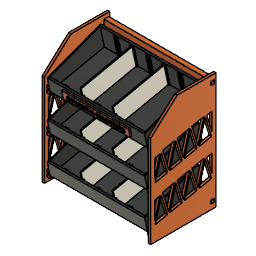
binstack-print-assembly.f3z (Autodesk Fusion 360 design; units mm, degrees)
part number: 2026-08-18-20-33-43-765
part number: 2026-08-18-20-33-45-073
part number: 2026-08-18-20-33-45-486
part number: 2026-08-18-20-33-45-986
part number: 2026-08-18-20-33-46-975
part number: 2026-08-18-20-33-47-360
part number: 2026-08-18-20-33-47-431
Autodesk Fusion 360 part; units mm, degrees
sketch "Sketch1" plane through (0, 0, 0) normal (1, 0, 0) x (0, 0, -1) in component "Боковина левая"
  line L0 (0, 15) -> (0, 150)
  line L1 (0, 150) -> (-240, 150)
  line L2 (-240, 150) -> (-240, 70)
  line L3 (-240, 70) -> (-190, 15)
  line L4 (-190, 15) -> (0, 15)
extrude "Extrude1" add sketch "Sketch1" along normal blind 5 from surface at 3 makes body 1 in component "Боковина левая"
sketch "Sketch2" plane through (0, 0, 0) normal (1, 0, 0) x (0, 0, -1) in component "Боковина левая"
  line L0 (-9, 20) -> (-35.5696, 145)
  line L1 (-35.5696, 145) -> (-41.5696, 145)
  line L2 (-41.5696, 145) -> (-15, 20)
  line L3 (-15, 20) -> (-9, 20)
extrude "Extrude2" add sketch "Sketch2" along normal blind 6 from surface at 8 separate body makes body 2 in component "Боковина левая"
sketch "Sketch3" plane through (0, 0, 0) normal (1, 0, 0) x (0, 0, -1) in component "Боковина левая"
  line L0 (-18.2, 20) -> (-44.7696, 145)
  line L1 (-44.7696, 145) -> (-49.7696, 145)
  line L2 (-49.7696, 145) -> (-23.2, 20)
  line L3 (-23.2, 20) -> (-18.2, 20)
extrude "Extrude3" add sketch "Sketch3" along normal blind 6 from surface at 8 separate body makes body 3 in component "Боковина левая"
sketch "Sketch4" plane through (0, 0, 0) normal (1, 0, 0) x (0, 0, -1) in component "Боковина левая"
  line L0 (-16.2753, 26) -> (-17.2753, 28)
  line L1 (-17.2753, 28) -> (-18.3381, 31)
  line L2 (-18.3381, 31) -> (-17.7632, 33)
  line L3 (-17.7632, 33) -> (-16.2753, 26)
extrude "Extrude4" add sketch "Sketch4" along normal blind 6 from surface at 8 separate body makes body 4 in component "Боковина левая"
sketch "Sketch5" plane through (0, 0, 0) normal (1, 0, 0) x (0, 0, -1) in component "Боковина левая"
  line L0 (-84, 20) -> (-110.5696, 145)
  line L1 (-110.5696, 145) -> (-116.5696, 145)
  line L2 (-116.5696, 145) -> (-90, 20)
  line L3 (-90, 20) -> (-84, 20)
extrude "Extrude5" add sketch "Sketch5" along normal blind 6 from surface at 8 separate body makes body 5 in component "Боковина левая"
sketch "Sketch6" plane through (0, 0, 0) normal (1, 0, 0) x (0, 0, -1) in component "Боковина левая"
  line L0 (-93.2, 20) -> (-119.7696, 145)
  line L1 (-119.7696, 145) -> (-124.7696, 145)
  line L2 (-124.7696, 145) -> (-98.2, 20)
  line L3 (-98.2, 20) -> (-93.2, 20)
extrude "Extrude6" add sketch "Sketch6" along normal blind 6 from surface at 8 separate body makes body 6 in component "Боковина левая"
sketch "Sketch7" plane through (0, 0, 0) normal (1, 0, 0) x (0, 0, -1) in component "Боковина левая"
  line L0 (-91.2753, 26) -> (-92.2753, 28)
  line L1 (-92.2753, 28) -> (-93.3381, 31)
  line L2 (-93.3381, 31) -> (-92.7632, 33)
  line L3 (-92.7632, 33) -> (-91.2753, 26)
extrude "Extrude7" add sketch "Sketch7" along normal blind 6 from surface at 8 separate body makes body 7 in component "Боковина левая"
sketch "Sketch8" plane through (0, 0, 0) normal (1, 0, 0) x (0, 0, -1) in component "Боковина левая"
  line L0 (-159, 20) -> (-185.5696, 145)
  line L1 (-185.5696, 145) -> (-191.5696, 145)
  line L2 (-191.5696, 145) -> (-165, 20)
  line L3 (-165, 20) -> (-159, 20)
extrude "Extrude8" add sketch "Sketch8" along normal blind 6 from surface at 8 separate body makes body 8 in component "Боковина левая"
sketch "Sketch9" plane through (0, 0, 0) normal (1, 0, 0) x (0, 0, -1) in component "Боковина левая"
  line L0 (-168.2, 20) -> (-194.7696, 145)
  line L1 (-194.7696, 145) -> (-199.7696, 145)
  line L2 (-199.7696, 145) -> (-173.2, 20)
  line L3 (-173.2, 20) -> (-168.2, 20)
extrude "Extrude9" add sketch "Sketch9" along normal blind 6 from surface at 8 separate body makes body 9 in component "Боковина левая"
sketch "Sketch10" plane through (0, 0, 0) normal (1, 0, 0) x (0, 0, -1) in component "Боковина левая"
  line L0 (-166.2753, 26) -> (-167.2753, 28)
  line L1 (-167.2753, 28) -> (-168.3381, 31)
  line L2 (-168.3381, 31) -> (-167.7632, 33)
  line L3 (-167.7632, 33) -> (-166.2753, 26)
extrude "Extrude10" add sketch "Sketch10" along normal blind 6 from surface at 8 separate body makes body 10 in component "Боковина левая"
combine "Combine1" operation add target body 1 tool bodies 2 3 4 5 6 7 8 9 10 in component "Боковина левая"
sketch "Sketch11" plane through (0, 0, 0) normal (1, 0, 0) x (0, 0, -1) in component "Боковина левая"
  line L0 (-10.5, 139.5) -> (-10.5, 146.5)
  line L1 (-10.5, 146.5) -> (-17.5, 146.5)
  line L2 (-17.5, 146.5) -> (-17.5, 139.5)
  line L3 (-17.5, 139.5) -> (-10.5, 139.5)
extrude "Extrude11" cut sketch "Sketch11" along normal blind 30 from surface at -2 bodies 1 in component "Боковина левая"
sketch "Sketch12" plane through (0, 0, 0) normal (1, 0, 0) x (0, 0, -1) in component "Боковина левая"
  line L0 (-222.5, 139.5) -> (-222.5, 146.5)
  line L1 (-222.5, 146.5) -> (-229.5, 146.5)
  line L2 (-229.5, 146.5) -> (-229.5, 139.5)
  line L3 (-229.5, 139.5) -> (-222.5, 139.5)
extrude "Extrude12" cut sketch "Sketch12" along normal blind 30 from surface at -2 bodies 1 in component "Боковина левая"
sketch "Sketch13" plane through (0, 0, 0) normal (1, 0, 0) x (0, 0, -1) in component "Боковина левая"
  line L0 (-31.2766, 24.6534) -> (-36.5785, 49.5966)
  line L1 (-36.5785, 49.5966) -> (-77.4649, 37.125)
  line L2 (-77.4649, 37.125) -> (-31.2766, 24.6534)
  line L3 (-37.7065, 54.9034) -> (-43.0083, 79.8466)
  line L4 (-43.0083, 79.8466) -> (-83.8948, 67.375)
  line L5 (-83.8948, 67.375) -> (-37.7065, 54.9034)
  line L6 (-44.1363, 85.1534) -> (-49.4382, 110.0966)
  line L7 (-49.4382, 110.0966) -> (-90.3246, 97.625)
  line L8 (-90.3246, 97.625) -> (-44.1363, 85.1534)
  line L9 (-50.5662, 115.4034) -> (-55.868, 140.3466)
  line L10 (-55.868, 140.3466) -> (-96.7545, 127.875)
  line L11 (-96.7545, 127.875) -> (-50.5662, 115.4034)
  line L12 (-81.1165, 39.7784) -> (-86.4183, 64.7216)
  line L13 (-86.4183, 64.7216) -> (-40.23, 52.25)
  line L14 (-40.23, 52.25) -> (-81.1165, 39.7784)
  line L15 (-87.5463, 70.0284) -> (-92.8482, 94.9716)
  line L16 (-92.8482, 94.9716) -> (-46.6599, 82.5)
  line L17 (-46.6599, 82.5) -> (-87.5463, 70.0284)
  line L18 (-93.9761, 100.2784) -> (-99.278, 125.2216)
  line L19 (-99.278, 125.2216) -> (-53.0897, 112.75)
  line L20 (-53.0897, 112.75) -> (-93.9761, 100.2784)
  line L21 (-38.7844, 23.5511) -> (-75.34, 23.5511)
  line L22 (-75.34, 23.5511) -> (-77.5658, 34.0228)
  line L23 (-77.5658, 34.0228) -> (-38.7844, 23.5511)
  line L24 (-63.8444, 141.4489) -> (-100.3999, 141.4489)
  line L25 (-100.3999, 141.4489) -> (-98.1741, 130.9772)
  line L26 (-98.1741, 130.9772) -> (-63.8444, 141.4489)
  line L27 (-106.2766, 24.6534) -> (-111.5785, 49.5966)
  line L28 (-111.5785, 49.5966) -> (-152.4649, 37.125)
  line L29 (-152.4649, 37.125) -> (-106.2766, 24.6534)
  line L30 (-112.7065, 54.9034) -> (-118.0083, 79.8466)
  line L31 (-118.0083, 79.8466) -> (-158.8948, 67.375)
  line L32 (-158.8948, 67.375) -> (-112.7065, 54.9034)
  line L33 (-119.1363, 85.1534) -> (-124.4382, 110.0966)
  line L34 (-124.4382, 110.0966) -> (-165.3246, 97.625)
  line L35 (-165.3246, 97.625) -> (-119.1363, 85.1534)
  line L36 (-125.5662, 115.4034) -> (-130.868, 140.3466)
  line L37 (-130.868, 140.3466) -> (-171.7545, 127.875)
  line L38 (-171.7545, 127.875) -> (-125.5662, 115.4034)
  line L39 (-156.1165, 39.7784) -> (-161.4183, 64.7216)
  line L40 (-161.4183, 64.7216) -> (-115.23, 52.25)
  line L41 (-115.23, 52.25) -> (-156.1165, 39.7784)
  line L42 (-162.5463, 70.0284) -> (-167.8482, 94.9716)
  line L43 (-167.8482, 94.9716) -> (-121.6599, 82.5)
  line L44 (-121.6599, 82.5) -> (-162.5463, 70.0284)
  line L45 (-168.9761, 100.2784) -> (-174.278, 125.2216)
  line L46 (-174.278, 125.2216) -> (-128.0897, 112.75)
  line L47 (-128.0897, 112.75) -> (-168.9761, 100.2784)
  line L48 (-113.7844, 23.5511) -> (-150.34, 23.5511)
  line L49 (-150.34, 23.5511) -> (-152.5658, 34.0228)
  line L50 (-152.5658, 34.0228) -> (-113.7844, 23.5511)
  line L51 (-138.8444, 141.4489) -> (-175.3999, 141.4489)
  line L52 (-175.3999, 141.4489) -> (-173.1741, 130.9772)
  line L53 (-173.1741, 130.9772) -> (-138.8444, 141.4489)
extrude "Extrude13" cut sketch "Sketch13" along normal blind 9 from surface at 1 bodies 1 in component "Боковина левая"
sketch "Sketch1 (2)" plane through (0, 0, 0) normal (1, 0, 0) x (0, 0, -1) in component "Боковина правая"
  line L0 (0, 15) -> (0, 150)
  line L1 (0, 150) -> (-240, 150)
  line L2 (-240, 150) -> (-240, 70)
  line L3 (-240, 70) -> (-190, 15)
  line L4 (-190, 15) -> (0, 15)
extrude "Extrude1'" add sketch "Sketch1 (2)" along normal blind 5 from surface at 6 separate body makes body 11 in component "Боковина правая"
sketch "Sketch2 (2)" plane through (0, 0, 0) normal (1, 0, 0) x (0, 0, -1) in component "Боковина правая"
  line L0 (-9, 20) -> (-35.5696, 145)
  line L1 (-35.5696, 145) -> (-41.5696, 145)
  line L2 (-41.5696, 145) -> (-15, 20)
  line L3 (-15, 20) -> (-9, 20)
extrude "Extrude2'" add sketch "Sketch2 (2)" along normal blind 6 separate body makes body 12 in component "Боковина правая"
sketch "Sketch3 (2)" plane through (0, 0, 0) normal (1, 0, 0) x (0, 0, -1) in component "Боковина правая"
  line L0 (-18.2, 20) -> (-44.7696, 145)
  line L1 (-44.7696, 145) -> (-49.7696, 145)
  line L2 (-49.7696, 145) -> (-23.2, 20)
  line L3 (-23.2, 20) -> (-18.2, 20)
extrude "Extrude3'" add sketch "Sketch3 (2)" along normal blind 6 separate body makes body 13 in component "Боковина правая"
sketch "Sketch4 (2)" plane through (0, 0, 0) normal (1, 0, 0) x (0, 0, -1) in component "Боковина правая"
  line L0 (-16.2753, 26) -> (-17.2753, 28)
  line L1 (-17.2753, 28) -> (-18.3381, 31)
  line L2 (-18.3381, 31) -> (-17.7632, 33)
  line L3 (-17.7632, 33) -> (-16.2753, 26)
extrude "Extrude4'" add sketch "Sketch4 (2)" along normal blind 6 separate body makes body 14 in component "Боковина правая"
sketch "Sketch5 (2)" plane through (0, 0, 0) normal (1, 0, 0) x (0, 0, -1) in component "Боковина правая"
  line L0 (-84, 20) -> (-110.5696, 145)
  line L1 (-110.5696, 145) -> (-116.5696, 145)
  line L2 (-116.5696, 145) -> (-90, 20)
  line L3 (-90, 20) -> (-84, 20)
extrude "Extrude5'" add sketch "Sketch5 (2)" along normal blind 6 separate body makes body 15 in component "Боковина правая"
sketch "Sketch6 (2)" plane through (0, 0, 0) normal (1, 0, 0) x (0, 0, -1) in component "Боковина правая"
  line L0 (-93.2, 20) -> (-119.7696, 145)
  line L1 (-119.7696, 145) -> (-124.7696, 145)
  line L2 (-124.7696, 145) -> (-98.2, 20)
  line L3 (-98.2, 20) -> (-93.2, 20)
extrude "Extrude6'" add sketch "Sketch6 (2)" along normal blind 6 separate body makes body 16 in component "Боковина правая"
sketch "Sketch7 (2)" plane through (0, 0, 0) normal (1, 0, 0) x (0, 0, -1) in component "Боковина правая"
  line L0 (-91.2753, 26) -> (-92.2753, 28)
  line L1 (-92.2753, 28) -> (-93.3381, 31)
  line L2 (-93.3381, 31) -> (-92.7632, 33)
  line L3 (-92.7632, 33) -> (-91.2753, 26)
extrude "Extrude7'" add sketch "Sketch7 (2)" along normal blind 6 separate body makes body 17 in component "Боковина правая"
sketch "Sketch8 (2)" plane through (0, 0, 0) normal (1, 0, 0) x (0, 0, -1) in component "Боковина правая"
  line L0 (-159, 20) -> (-185.5696, 145)
  line L1 (-185.5696, 145) -> (-191.5696, 145)
  line L2 (-191.5696, 145) -> (-165, 20)
  line L3 (-165, 20) -> (-159, 20)
extrude "Extrude8'" add sketch "Sketch8 (2)" along normal blind 6 separate body makes body 18 in component "Боковина правая"
sketch "Sketch9 (2)" plane through (0, 0, 0) normal (1, 0, 0) x (0, 0, -1) in component "Боковина правая"
  line L0 (-168.2, 20) -> (-194.7696, 145)
  line L1 (-194.7696, 145) -> (-199.7696, 145)
  line L2 (-199.7696, 145) -> (-173.2, 20)
  line L3 (-173.2, 20) -> (-168.2, 20)
extrude "Extrude9'" add sketch "Sketch9 (2)" along normal blind 6 separate body makes body 19 in component "Боковина правая"
sketch "Sketch10 (2)" plane through (0, 0, 0) normal (1, 0, 0) x (0, 0, -1) in component "Боковина правая"
  line L0 (-166.2753, 26) -> (-167.2753, 28)
  line L1 (-167.2753, 28) -> (-168.3381, 31)
  line L2 (-168.3381, 31) -> (-167.7632, 33)
  line L3 (-167.7632, 33) -> (-166.2753, 26)
extrude "Extrude10'" add sketch "Sketch10 (2)" along normal blind 6 separate body makes body 20 in component "Боковина правая"
combine "Combine1'" operation add target body 11 tool bodies 12 13 14 15 16 17 18 19 20 in component "Боковина правая"
sketch "Sketch11 (2)" plane through (0, 0, 0) normal (1, 0, 0) x (0, 0, -1) in component "Боковина правая"
  line L0 (-10.5, 139.5) -> (-10.5, 146.5)
  line L1 (-10.5, 146.5) -> (-17.5, 146.5)
  line L2 (-17.5, 146.5) -> (-17.5, 139.5)
  line L3 (-17.5, 139.5) -> (-10.5, 139.5)
extrude "Extrude11'" cut sketch "Sketch11 (2)" along normal blind 30 from surface at -2 bodies 11 in component "Боковина правая"
sketch "Sketch12 (2)" plane through (0, 0, 0) normal (1, 0, 0) x (0, 0, -1) in component "Боковина правая"
  line L0 (-222.5, 139.5) -> (-222.5, 146.5)
  line L1 (-222.5, 146.5) -> (-229.5, 146.5)
  line L2 (-229.5, 146.5) -> (-229.5, 139.5)
  line L3 (-229.5, 139.5) -> (-222.5, 139.5)
extrude "Extrude12'" cut sketch "Sketch12 (2)" along normal blind 30 from surface at -2 bodies 11 in component "Боковина правая"
sketch "Sketch13 (2)" plane through (0, 0, 0) normal (1, 0, 0) x (0, 0, -1) in component "Боковина правая"
  line L0 (-31.2766, 24.6534) -> (-36.5785, 49.5966)
  line L1 (-36.5785, 49.5966) -> (-77.4649, 37.125)
  line L2 (-77.4649, 37.125) -> (-31.2766, 24.6534)
  line L3 (-37.7065, 54.9034) -> (-43.0083, 79.8466)
  line L4 (-43.0083, 79.8466) -> (-83.8948, 67.375)
  line L5 (-83.8948, 67.375) -> (-37.7065, 54.9034)
  line L6 (-44.1363, 85.1534) -> (-49.4382, 110.0966)
  line L7 (-49.4382, 110.0966) -> (-90.3246, 97.625)
  line L8 (-90.3246, 97.625) -> (-44.1363, 85.1534)
  line L9 (-50.5662, 115.4034) -> (-55.868, 140.3466)
  line L10 (-55.868, 140.3466) -> (-96.7545, 127.875)
  line L11 (-96.7545, 127.875) -> (-50.5662, 115.4034)
  line L12 (-81.1165, 39.7784) -> (-86.4183, 64.7216)
  line L13 (-86.4183, 64.7216) -> (-40.23, 52.25)
  line L14 (-40.23, 52.25) -> (-81.1165, 39.7784)
  line L15 (-87.5463, 70.0284) -> (-92.8482, 94.9716)
  line L16 (-92.8482, 94.9716) -> (-46.6599, 82.5)
  line L17 (-46.6599, 82.5) -> (-87.5463, 70.0284)
  line L18 (-93.9761, 100.2784) -> (-99.278, 125.2216)
  line L19 (-99.278, 125.2216) -> (-53.0897, 112.75)
  line L20 (-53.0897, 112.75) -> (-93.9761, 100.2784)
  line L21 (-38.7844, 23.5511) -> (-75.34, 23.5511)
  line L22 (-75.34, 23.5511) -> (-77.5658, 34.0228)
  line L23 (-77.5658, 34.0228) -> (-38.7844, 23.5511)
  line L24 (-63.8444, 141.4489) -> (-100.3999, 141.4489)
  line L25 (-100.3999, 141.4489) -> (-98.1741, 130.9772)
  line L26 (-98.1741, 130.9772) -> (-63.8444, 141.4489)
  line L27 (-106.2766, 24.6534) -> (-111.5785, 49.5966)
  line L28 (-111.5785, 49.5966) -> (-152.4649, 37.125)
  line L29 (-152.4649, 37.125) -> (-106.2766, 24.6534)
  line L30 (-112.7065, 54.9034) -> (-118.0083, 79.8466)
  line L31 (-118.0083, 79.8466) -> (-158.8948, 67.375)
  line L32 (-158.8948, 67.375) -> (-112.7065, 54.9034)
  line L33 (-119.1363, 85.1534) -> (-124.4382, 110.0966)
  line L34 (-124.4382, 110.0966) -> (-165.3246, 97.625)
  line L35 (-165.3246, 97.625) -> (-119.1363, 85.1534)
  line L36 (-125.5662, 115.4034) -> (-130.868, 140.3466)
  line L37 (-130.868, 140.3466) -> (-171.7545, 127.875)
  line L38 (-171.7545, 127.875) -> (-125.5662, 115.4034)
  line L39 (-156.1165, 39.7784) -> (-161.4183, 64.7216)
  line L40 (-161.4183, 64.7216) -> (-115.23, 52.25)
  line L41 (-115.23, 52.25) -> (-156.1165, 39.7784)
  line L42 (-162.5463, 70.0284) -> (-167.8482, 94.9716)
  line L43 (-167.8482, 94.9716) -> (-121.6599, 82.5)
  line L44 (-121.6599, 82.5) -> (-162.5463, 70.0284)
  line L45 (-168.9761, 100.2784) -> (-174.278, 125.2216)
  line L46 (-174.278, 125.2216) -> (-128.0897, 112.75)
  line L47 (-128.0897, 112.75) -> (-168.9761, 100.2784)
  line L48 (-113.7844, 23.5511) -> (-150.34, 23.5511)
  line L49 (-150.34, 23.5511) -> (-152.5658, 34.0228)
  line L50 (-152.5658, 34.0228) -> (-113.7844, 23.5511)
  line L51 (-138.8444, 141.4489) -> (-175.3999, 141.4489)
  line L52 (-175.3999, 141.4489) -> (-173.1741, 130.9772)
  line L53 (-173.1741, 130.9772) -> (-138.8444, 141.4489)
extrude "Extrude13'" cut sketch "Sketch13 (2)" along normal blind 9 from surface at 4 bodies 11 in component "Боковина правая"
sketch "Sketch1 (3)" plane through (0, 0, 0) normal (0, 0, 1) x (1, 0, 0) in component "Лоток"
  line L0 (-6, 0) -> (207, 0)
  line L1 (207, 0) -> (207, 117)
  line L2 (207, 117) -> (-6, 117)
  line L3 (-6, 117) -> (-6, 0)
extrude "Extrude1''" add sketch "Sketch1 (3)" along normal blind 2.4 separate body makes body 21 in component "Лоток"
sketch "Sketch2 (3)" plane through (0, 0, 0) normal (0, 0, 1) x (1, 0, 0) in component "Лоток"
  line L0 (0, 0) -> (201, 0)
  line L1 (201, 0) -> (201, 4)
  line L2 (201, 4) -> (0, 4)
  line L3 (0, 4) -> (0, 0)
extrude "Extrude2''" add sketch "Sketch2 (3)" along normal blind 28 separate body makes body 22 in component "Лоток"
sketch "Sketch3 (3)" plane through (0, 0, 0) normal (0, 0, 1) x (1, 0, 0) in component "Лоток"
  line L0 (0, 113) -> (201, 113)
  line L1 (201, 113) -> (201, 117)
  line L2 (201, 117) -> (0, 117)
  line L3 (0, 117) -> (0, 113)
extrude "Extrude3''" add sketch "Sketch3 (3)" along normal blind 45 separate body makes body 23 in component "Лоток"
sketch "Sketch4 (3)" plane through (0, 0, 0) normal (1, 0, 0) x (0, 0, -1) in component "Лоток"
  line L0 (0, 0) -> (0, 117)
  line L1 (0, 117) -> (-45, 117)
  line L2 (-45, 117) -> (-28, 0)
  line L3 (-28, 0) -> (0, 0)
extrude "Extrude4''" add sketch "Sketch4 (3)" along normal blind 2 separate body makes body 24 in component "Лоток"
sketch "Sketch5 (3)" plane through (0, 0, 0) normal (1, 0, 0) x (0, 0, -1) in component "Лоток"
  line L0 (0, 0) -> (0, 117)
  line L1 (0, 117) -> (-45, 117)
  line L2 (-45, 117) -> (-28, 0)
  line L3 (-28, 0) -> (0, 0)
extrude "Extrude5''" add sketch "Sketch5 (3)" along normal blind 2 from surface at 199 separate body makes body 25 in component "Лоток"
sketch "Sketch6 (3)" plane through (0, 0, 0) normal (0, 0, 1) x (1, 0, 0) in component "Лоток"
  line L0 (31.4, 4) -> (33.4, 4)
  line L1 (33.4, 4) -> (33.4, 6)
  line L2 (33.4, 6) -> (31.4, 6)
  line L3 (31.4, 6) -> (31.4, 4)
extrude "Extrude6''" add sketch "Sketch6 (3)" along normal blind 25.6 from surface at 2.4 separate body makes body 26 in component "Лоток"
sketch "Sketch7 (3)" plane through (0, 0, 0) normal (0, 0, 1) x (1, 0, 0) in component "Лоток"
  line L0 (31.4, 111) -> (33.4, 111)
  line L1 (33.4, 111) -> (33.4, 113)
  line L2 (33.4, 113) -> (31.4, 113)
  line L3 (31.4, 113) -> (31.4, 111)
extrude "Extrude7''" add sketch "Sketch7 (3)" along normal blind 42.6 from surface at 2.4 separate body makes body 27 in component "Лоток"
sketch "Sketch8 (3)" plane through (0, 0, 0) normal (0, 0, 1) x (1, 0, 0) in component "Лоток"
  line L0 (36.6, 4) -> (38.6, 4)
  line L1 (38.6, 4) -> (38.6, 6)
  line L2 (38.6, 6) -> (36.6, 6)
  line L3 (36.6, 6) -> (36.6, 4)
extrude "Extrude8''" add sketch "Sketch8 (3)" along normal blind 25.6 from surface at 2.4 separate body makes body 28 in component "Лоток"
sketch "Sketch9 (3)" plane through (0, 0, 0) normal (0, 0, 1) x (1, 0, 0) in component "Лоток"
  line L0 (36.6, 111) -> (38.6, 111)
  line L1 (38.6, 111) -> (38.6, 113)
  line L2 (38.6, 113) -> (36.6, 113)
  line L3 (36.6, 113) -> (36.6, 111)
extrude "Extrude9''" add sketch "Sketch9 (3)" along normal blind 42.6 from surface at 2.4 separate body makes body 29 in component "Лоток"
sketch "Sketch10 (3)" plane through (0, 0, 0) normal (0, 0, 1) x (1, 0, 0) in component "Лоток"
  line L0 (64.4, 4) -> (66.4, 4)
  line L1 (66.4, 4) -> (66.4, 6)
  line L2 (66.4, 6) -> (64.4, 6)
  line L3 (64.4, 6) -> (64.4, 4)
extrude "Extrude10''" add sketch "Sketch10 (3)" along normal blind 25.6 from surface at 2.4 separate body makes body 30 in component "Лоток"
sketch "Sketch11 (3)" plane through (0, 0, 0) normal (0, 0, 1) x (1, 0, 0) in component "Лоток"
  line L0 (64.4, 111) -> (66.4, 111)
  line L1 (66.4, 111) -> (66.4, 113)
  line L2 (66.4, 113) -> (64.4, 113)
  line L3 (64.4, 113) -> (64.4, 111)
extrude "Extrude11''" add sketch "Sketch11 (3)" along normal blind 42.6 from surface at 2.4 separate body makes body 31 in component "Лоток"
sketch "Sketch12 (3)" plane through (0, 0, 0) normal (0, 0, 1) x (1, 0, 0) in component "Лоток"
  line L0 (69.6, 4) -> (71.6, 4)
  line L1 (71.6, 4) -> (71.6, 6)
  line L2 (71.6, 6) -> (69.6, 6)
  line L3 (69.6, 6) -> (69.6, 4)
extrude "Extrude12''" add sketch "Sketch12 (3)" along normal blind 25.6 from surface at 2.4 separate body makes body 32 in component "Лоток"
sketch "Sketch13 (3)" plane through (0, 0, 0) normal (0, 0, 1) x (1, 0, 0) in component "Лоток"
  line L0 (69.6, 111) -> (71.6, 111)
  line L1 (71.6, 111) -> (71.6, 113)
  line L2 (71.6, 113) -> (69.6, 113)
  line L3 (69.6, 113) -> (69.6, 111)
extrude "Extrude13''" add sketch "Sketch13 (3)" along normal blind 42.6 from surface at 2.4 separate body makes body 33 in component "Лоток"
sketch "Sketch14" plane through (0, 0, 0) normal (0, 0, 1) x (1, 0, 0) in component "Лоток"
  line L0 (97.4, 4) -> (99.4, 4)
  line L1 (99.4, 4) -> (99.4, 6)
  line L2 (99.4, 6) -> (97.4, 6)
  line L3 (97.4, 6) -> (97.4, 4)
extrude "Extrude14" add sketch "Sketch14" along normal blind 25.6 from surface at 2.4 separate body makes body 34 in component "Лоток"
sketch "Sketch15" plane through (0, 0, 0) normal (0, 0, 1) x (1, 0, 0) in component "Лоток"
  line L0 (97.4, 111) -> (99.4, 111)
  line L1 (99.4, 111) -> (99.4, 113)
  line L2 (99.4, 113) -> (97.4, 113)
  line L3 (97.4, 113) -> (97.4, 111)
extrude "Extrude15" add sketch "Sketch15" along normal blind 42.6 from surface at 2.4 separate body makes body 35 in component "Лоток"
sketch "Sketch16" plane through (0, 0, 0) normal (0, 0, 1) x (1, 0, 0) in component "Лоток"
  line L0 (102.6, 4) -> (104.6, 4)
  line L1 (104.6, 4) -> (104.6, 6)
  line L2 (104.6, 6) -> (102.6, 6)
  line L3 (102.6, 6) -> (102.6, 4)
extrude "Extrude16" add sketch "Sketch16" along normal blind 25.6 from surface at 2.4 separate body makes body 36 in component "Лоток"
sketch "Sketch17" plane through (0, 0, 0) normal (0, 0, 1) x (1, 0, 0) in component "Лоток"
  line L0 (102.6, 111) -> (104.6, 111)
  line L1 (104.6, 111) -> (104.6, 113)
  line L2 (104.6, 113) -> (102.6, 113)
  line L3 (102.6, 113) -> (102.6, 111)
extrude "Extrude17" add sketch "Sketch17" along normal blind 42.6 from surface at 2.4 separate body makes body 37 in component "Лоток"
sketch "Sketch18" plane through (0, 0, 0) normal (0, 0, 1) x (1, 0, 0) in component "Лоток"
  line L0 (130.4, 4) -> (132.4, 4)
  line L1 (132.4, 4) -> (132.4, 6)
  line L2 (132.4, 6) -> (130.4, 6)
  line L3 (130.4, 6) -> (130.4, 4)
extrude "Extrude18" add sketch "Sketch18" along normal blind 25.6 from surface at 2.4 separate body makes body 38 in component "Лоток"
sketch "Sketch19" plane through (0, 0, 0) normal (0, 0, 1) x (1, 0, 0) in component "Лоток"
  line L0 (130.4, 111) -> (132.4, 111)
  line L1 (132.4, 111) -> (132.4, 113)
  line L2 (132.4, 113) -> (130.4, 113)
  line L3 (130.4, 113) -> (130.4, 111)
extrude "Extrude19" add sketch "Sketch19" along normal blind 42.6 from surface at 2.4 separate body makes body 39 in component "Лоток"
sketch "Sketch20" plane through (0, 0, 0) normal (0, 0, 1) x (1, 0, 0) in component "Лоток"
  line L0 (135.6, 4) -> (137.6, 4)
  line L1 (137.6, 4) -> (137.6, 6)
  line L2 (137.6, 6) -> (135.6, 6)
  line L3 (135.6, 6) -> (135.6, 4)
extrude "Extrude20" add sketch "Sketch20" along normal blind 25.6 from surface at 2.4 separate body makes body 40 in component "Лоток"
sketch "Sketch21" plane through (0, 0, 0) normal (0, 0, 1) x (1, 0, 0) in component "Лоток"
  line L0 (135.6, 111) -> (137.6, 111)
  line L1 (137.6, 111) -> (137.6, 113)
  line L2 (137.6, 113) -> (135.6, 113)
  line L3 (135.6, 113) -> (135.6, 111)
extrude "Extrude21" add sketch "Sketch21" along normal blind 42.6 from surface at 2.4 separate body makes body 41 in component "Лоток"
sketch "Sketch22" plane through (0, 0, 0) normal (0, 0, 1) x (1, 0, 0) in component "Лоток"
  line L0 (163.4, 4) -> (165.4, 4)
  line L1 (165.4, 4) -> (165.4, 6)
  line L2 (165.4, 6) -> (163.4, 6)
  line L3 (163.4, 6) -> (163.4, 4)
extrude "Extrude22" add sketch "Sketch22" along normal blind 25.6 from surface at 2.4 separate body makes body 42 in component "Лоток"
sketch "Sketch23" plane through (0, 0, 0) normal (0, 0, 1) x (1, 0, 0) in component "Лоток"
  line L0 (163.4, 111) -> (165.4, 111)
  line L1 (165.4, 111) -> (165.4, 113)
  line L2 (165.4, 113) -> (163.4, 113)
  line L3 (163.4, 113) -> (163.4, 111)
extrude "Extrude23" add sketch "Sketch23" along normal blind 42.6 from surface at 2.4 separate body makes body 43 in component "Лоток"
sketch "Sketch24" plane through (0, 0, 0) normal (0, 0, 1) x (1, 0, 0) in component "Лоток"
  line L0 (168.6, 4) -> (170.6, 4)
  line L1 (170.6, 4) -> (170.6, 6)
  line L2 (170.6, 6) -> (168.6, 6)
  line L3 (168.6, 6) -> (168.6, 4)
extrude "Extrude24" add sketch "Sketch24" along normal blind 25.6 from surface at 2.4 separate body makes body 44 in component "Лоток"
sketch "Sketch25" plane through (0, 0, 0) normal (0, 0, 1) x (1, 0, 0) in component "Лоток"
  line L0 (168.6, 111) -> (170.6, 111)
  line L1 (170.6, 111) -> (170.6, 113)
  line L2 (170.6, 113) -> (168.6, 113)
  line L3 (168.6, 113) -> (168.6, 111)
extrude "Extrude25" add sketch "Sketch25" along normal blind 42.6 from surface at 2.4 separate body makes body 45 in component "Лоток"
combine "Combine1''" operation add target body 21 tool bodies 22 23 24 25 26 27 28 29 30 31 32 33 34 35 36 37 38 39 40 41 42 43 44 45 in component "Лоток"
sketch "Sketch1 (4)" plane through (0, 0, 0) normal (0, 0, 1) x (1, 0, 0) in component "Планка логотипа"
  line L0 (0, 0) -> (120, 0)
  dimension "d154" = 8
  text T0 "GIVANTA MASTERS" font "Arial Black" height 8 align centre spacing 1 along the path L0 letters at x, y, angle (-0.6003, 12.3001, 0) (8.7094, 12.3001, 0) (13.0587, 12.3001, 0) (21.7626, 12.3001, 0) (30.4884, 12.3001, 0) (39.7981, 12.3001, 0) (47.869, 12.3001, 0) (56.5948, 12.3001, 0) (60.322, 12.3001, 0) (70.8704, 12.3001, 0) (79.5962, 12.3001, 0) (87.6671, 12.3001, 0) (95.7381, 12.3001, 0) (103.809, 12.3001, 0) (112.5293, 12.3001, 0)
extrude "Extrude1'''" add sketch "Sketch1 (4)" along normal blind 0.8 separate body text T0 makes body 46 at (97.377, 3.7963, 0) makes body 47 at (61.7881, 4.7003, 0) makes body 48 at (28.3147, 3.6835, 0) makes body 49 at (7.3379, 2.8704, 0) makes body 50 at (38.1974, 3.8581, 0) makes body 51 at (77.4225, 3.6835, 0) makes body 52 at (105.4879, 3.749, 0) makes body 53 at (91.2688, 4.0164, 0) makes body 54 at (54.4211, 3.6835, 0) makes body 55 at (15.5562, 3.4143, 0) makes body 56 at (10.452, 5.3333, 0) makes body 57 at (43.3997, 4.0164, 0) makes body 58 at (85.0771, 4.1947, 0) makes body 59 at (118.0102, 4.1947, 0) in component "Планка логотипа"
sketch "Sketch2 (4)" plane through (0, 0, 0) normal (0, 0, 1) x (1, 0, 0) in component "Планка логотипа"
  line L0 (-9.0873, -4.6364) -> (129.1746, -4.6364)
  line L1 (129.1746, -4.6364) -> (129.1746, 12.6364)
  line L2 (129.1746, 12.6364) -> (-9.0873, 12.6364)
  line L3 (-9.0873, 12.6364) -> (-9.0873, -4.6364)
extrude "Extrude2'''" add sketch "Sketch2 (4)" along normal blind 3 from surface at -3 separate body makes body 60 in component "Планка логотипа"
sketch "Sketch1 (5)" plane through (0, 0, 0) normal (0, 0, 1) x (1, 0, 0) in component "Перегородка"
  line L0 (0, 0) -> (2.4, 0)
  line L1 (2.4, 0) -> (2.4, 109)
  line L2 (2.4, 109) -> (0, 109)
  line L3 (0, 109) -> (0, 0)
extrude "Extrude1''''" add sketch "Sketch1 (5)" along normal blind 40 separate body makes body 61 in component "Перегородка"
sketch "Sketch1 (6)" plane through (0, 0, 0) normal (0, 0, 1) x (1, 0, 0) in component "Штанга"
  line L0 (0, 0) -> (214, 0)
  line L1 (214, 0) -> (214, 10)
  line L2 (214, 10) -> (0, 10)
  line L3 (0, 10) -> (0, 0)
extrude "Extrude1'''''" add sketch "Sketch1 (6)" along normal blind 12 separate body makes body 62 in component "Штанга"
sketch "Sketch2 (5)" plane through (0, 0, 0) normal (0, 0, 1) x (1, 0, 0) in component "Штанга"
  line L0 (-5, 2) -> (0, 2)
  line L1 (0, 2) -> (0, 8)
  line L2 (0, 8) -> (-5, 8)
  line L3 (-5, 8) -> (-5, 2)
extrude "Extrude2''''" add sketch "Sketch2 (5)" along normal blind 6 from surface at 3 separate body makes body 63 in component "Штанга"
sketch "Sketch3 (4)" plane through (0, 0, 0) normal (0, 0, 1) x (1, 0, 0) in component "Штанга"
  line L0 (214, 2) -> (219, 2)
  line L1 (219, 2) -> (219, 8)
  line L2 (219, 8) -> (214, 8)
  line L3 (214, 8) -> (214, 2)
extrude "Extrude3'''" add sketch "Sketch3 (4)" along normal blind 6 from surface at 3 separate body makes body 64 in component "Штанга"
combine "Combine1'''" operation add target body 62 tool bodies 63 64 in component "Штанга"
component "Боковина левая" placed x (1, 0, 0) y (0, 1, 0) z (0, 0, 1) at (0, 0, 0)
component "Боковина правая" placed x (1, 0, 0) y (0, 1, 0) z (0, 0, 1) at (216, 0, 0)
component "Лоток" placed x (1, 0, 0) y (0, 0.978148, 0.207912) z (0, -0.207912, 0.978148) at (14.5, 20, 15)
component "Перегородка" placed x (1, 0, 0) y (0, 0.978148, 0.207912) z (0, -0.207912, 0.978148) at (81.3, 23.4136, 18.1792)
component "Штанга" placed x (1, 0, 0) y (0, 1, 0) z (0, 0, 1) at (8, 138, 8)
component "Лоток" placed x (1, 0, 0) y (0, 0.978148, 0.207912) z (0, -0.207912, 0.978148) at (14.5, 20, 90)
component "Лоток" placed x (1, 0, 0) y (0, 0.978148, 0.207912) z (0, -0.207912, 0.978148) at (14.5, 20, 165)
component "Перегородка" placed x (1, 0, 0) y (0, 0.978148, 0.207912) z (0, -0.207912, 0.978148) at (147.3, 23.4136, 18.1792)
component "Перегородка" placed x (1, 0, 0) y (0, 0.978148, 0.207912) z (0, -0.207912, 0.978148) at (81.3, 23.4136, 93.1792)
component "Перегородка" placed x (1, 0, 0) y (0, 0.978148, 0.207912) z (0, -0.207912, 0.978148) at (147.3, 23.4136, 93.1792)
component "Перегородка" placed x (1, 0, 0) y (0, 0.978148, 0.207912) z (0, -0.207912, 0.978148) at (81.3, 23.4136, 168.1792)
component "Перегородка" placed x (1, 0, 0) y (0, 0.978148, 0.207912) z (0, -0.207912, 0.978148) at (147.3, 23.4136, 168.1792)
component "Штанга" placed x (1, 0, 0) y (0, 1, 0) z (0, 0, 1) at (8, 138, 220)
component "Планка логотипа" placed x (1, 0, 0) y (0, -0.207912, 0.978148) z (0, -0.978148, -0.207912) at (54.9563, 15.062, 173.8021)
equation "d155 = 'GIVANTA MASTERS'"
named bodies: "Тело", "Логотип (2-й цвет)", "Логотип", "Логотип (1)", "Логотип (2)", "Логотип (3)", "Логотип (4)", "Логотип (5)", "Логотип (6)", "Логотип (7)", "Логотип (8)", "Логотип (9)", "Логотип (10)", "Логотип (11)", "Логотип (12)"
